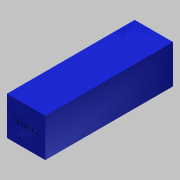
# Autodesk Inventor part: Container 2 2 5 generic
Saved by Autodesk Inventor 2015 (Build 190159000, 159)
## iProperties
Created: 2015-03-07
Part Number: Container 2 2 5 generic
Material: Generic
Document SubType Name: Modeling
Designer: Vukica
Density: 1 g/cm^3
Appearance: Blue - Wall Paint - Glossy
Author: Vukica
Autodesk Inventor part; units mm, degrees
ref_plane "YZ Plane" through (0, 0, 0) normal (1, 0, 0) x (0, 1, 0)
ref_plane "XZ Plane" through (0, 0, 0) normal (0, 1, 0) x (-1, 0, 0)
ref_plane "XY Plane" through (0, 0, 0) normal (0, 0, 1) x (1, 0, 0)
sketch "Sketch1" plane through (0, 0, 0) normal (0, 0, 1) x (1, 0, 0)
  line L0 (0, 0) -> (38.1, 0)
  line L1 (38.1, 0) -> (38.1, 38.1)
  line L2 (38.1, 38.1) -> (0, 38.1)
  line L3 (0, 38.1) -> (0, 0)
  dimension "d0" = 38.1
  dimension "d1" = 38.1
  constraints: 8 end point, 2 parallel, 1 horizontal, 1 perpendicular
  measures "d0" distance of L1.end L2.end
  measures "d1" distance of L2.end L0.start
extrude "Extrusion1" add sketch "Sketch1" along normal blind 127
sketch "Sketch2" plane through (0, 0, 127) normal (0, 0, 1) x (1, 0, 0)
  line L0 (5.3755, 22.1024) -> (51.7707, 22.1024) construction
  line L1 (51.7707, 22.1024) -> (51.7707, -10.5224) construction
  line L2 (51.7707, -10.5224) -> (5.3755, -10.5224) construction
  line L3 (5.3755, -10.5224) -> (5.3755, 22.1024) construction
  spline S0 degree 2 poles (8.0184, 16.8331) (7.4792, 16.8331) (6.5858, 17.1624) (6.2647, 17.4959) knots 0 0 0 1 2 2 2
  spline S1 degree 2 poles (6.2647, 17.4959) (5.9436, 17.8334) (5.6019, 18.8297) (5.6019, 19.476) knots 0 0 0 1 2 2 2
  spline S2 degree 2 poles (5.6019, 19.476) (5.6019, 20.0894) (5.9478, 21.0609) (6.2689, 21.4067) knots 0 0 0 1 2 2 2
  spline S3 degree 2 poles (6.2689, 21.4067) (6.5776, 21.7402) (7.4833, 22.1024) (8.0226, 22.1024) knots 0 0 0 1 2 2 2
  spline S4 degree 2 poles (8.0226, 22.1024) (8.2819, 22.1024) (8.7512, 22.0283) (8.9653, 21.9625) knots 0 0 0 1 2 2 2
  spline S5 degree 2 poles (8.9653, 21.9625) (9.1382, 21.9131) (9.5581, 21.7319) (9.6857, 21.6661) knots 0 0 0 1 2 2 2
  line L4 (9.6857, 21.6661) -> (9.6857, 20.851)
  line L5 (9.6857, 20.851) -> (9.6281, 20.851)
  spline S6 degree 2 poles (9.6281, 20.851) (9.5005, 20.9621) (9.2329, 21.1638) (8.9859, 21.2791) knots 0 0 0 1 2 2 2
  spline S7 degree 2 poles (8.9859, 21.2791) (8.78, 21.382) (8.249, 21.5179) (7.9443, 21.5179) knots 0 0 0 1 2 2 2
  spline S8 degree 2 poles (7.9443, 21.5179) (7.2116, 21.5179) (6.3059, 20.4146) (6.3059, 19.4966) knots 0 0 0 1 2 2 2
  spline S9 degree 2 poles (6.3059, 19.4966) (6.3059, 18.9861) (6.5447, 18.2204) (6.7711, 17.9569) knots 0 0 0 1 2 2 2
  spline S10 degree 2 poles (6.7711, 17.9569) (6.9893, 17.6935) (7.6068, 17.4176) (7.9937, 17.4176) knots 0 0 0 1 2 2 2
  spline S11 degree 2 poles (7.9937, 17.4176) (8.2778, 17.4176) (8.8459, 17.5) (9.0394, 17.5823) knots 0 0 0 1 2 2 2
  line L6 (9.0394, 17.5823) -> (9.0394, 18.8955)
  line L7 (9.0394, 18.8955) -> (7.862, 18.8955)
  line L8 (7.862, 18.8955) -> (7.862, 19.4883)
  line L9 (7.862, 19.4883) -> (9.7063, 19.4883)
  line L10 (9.7063, 19.4883) -> (9.7063, 17.2694)
  spline S12 degree 2 poles (9.7063, 17.2694) (9.5787, 17.2118) (9.1423, 17.0348) (8.9571, 16.9813) knots 0 0 0 1 2 2 2
  spline S13 degree 2 poles (8.9571, 16.9813) (8.7059, 16.9072) (8.3025, 16.8331) (8.0184, 16.8331) knots 0 0 0 1 2 2 2
  line L11 (10.5543, 16.9319) -> (10.5543, 22.0119)
  line L12 (10.5543, 22.0119) -> (13.7324, 22.0119)
  line L13 (13.7324, 22.0119) -> (13.7324, 21.4108)
  line L14 (13.7324, 21.4108) -> (11.2295, 21.4108)
  line L15 (11.2295, 21.4108) -> (11.2295, 20.0194)
  line L16 (11.2295, 20.0194) -> (13.5636, 20.0194)
  line L17 (13.5636, 20.0194) -> (13.5636, 19.4184)
  line L18 (13.5636, 19.4184) -> (11.2295, 19.4184)
  line L19 (11.2295, 19.4184) -> (11.2295, 17.5329)
  line L20 (11.2295, 17.5329) -> (13.7324, 17.5329)
  line L21 (13.7324, 17.5329) -> (13.7324, 16.9319)
  line L22 (13.7324, 16.9319) -> (10.5543, 16.9319)
  line L23 (18.1085, 16.9319) -> (17.351, 16.9319)
  line L24 (17.351, 16.9319) -> (15.1033, 21.312)
  line L25 (15.1033, 21.312) -> (15.1033, 16.9319)
  line L26 (15.1033, 16.9319) -> (14.4734, 16.9319)
  line L27 (14.4734, 16.9319) -> (14.4734, 22.0119)
  line L28 (14.4734, 22.0119) -> (15.4326, 22.0119)
  line L29 (15.4326, 22.0119) -> (17.4786, 17.9899)
  line L30 (17.4786, 17.9899) -> (17.4786, 22.0119)
  line L31 (17.4786, 22.0119) -> (18.1085, 22.0119)
  line L32 (18.1085, 22.0119) -> (18.1085, 16.9319)
  line L33 (19.1376, 16.9319) -> (19.1376, 22.0119)
  line L34 (19.1376, 22.0119) -> (22.3157, 22.0119)
  line L35 (22.3157, 22.0119) -> (22.3157, 21.4108)
  line L36 (22.3157, 21.4108) -> (19.8128, 21.4108)
  line L37 (19.8128, 21.4108) -> (19.8128, 20.0194)
  line L38 (19.8128, 20.0194) -> (22.1469, 20.0194)
  line L39 (22.1469, 20.0194) -> (22.1469, 19.4184)
  line L40 (22.1469, 19.4184) -> (19.8128, 19.4184)
  line L41 (19.8128, 19.4184) -> (19.8128, 17.5329)
  line L42 (19.8128, 17.5329) -> (22.3157, 17.5329)
  line L43 (22.3157, 17.5329) -> (22.3157, 16.9319)
  line L44 (22.3157, 16.9319) -> (19.1376, 16.9319)
  line L45 (26.9882, 16.9319) -> (26.1113, 16.9319)
  line L46 (26.1113, 16.9319) -> (24.5058, 18.9532)
  line L47 (24.5058, 18.9532) -> (23.7319, 18.9532)
  line L48 (23.7319, 18.9532) -> (23.7319, 16.9319)
  line L49 (23.7319, 16.9319) -> (23.0567, 16.9319)
  line L50 (23.0567, 16.9319) -> (23.0567, 22.0119)
  line L51 (23.0567, 22.0119) -> (24.3658, 22.0119)
  spline S14 degree 2 poles (24.3658, 22.0119) (24.8022, 22.0119) (25.3909, 21.9172) (25.6585, 21.7443) knots 0 0 0 1 2 2 2
  spline S15 degree 2 poles (25.6585, 21.7443) (25.9261, 21.5714) (26.2348, 21.0321) (26.2348, 20.6328) knots 0 0 0 1 2 2 2
  spline S16 degree 2 poles (26.2348, 20.6328) (26.2348, 20.077) (25.6667, 19.3237) (25.1809, 19.1425) knots 0 0 0 1 2 2 2
  line L52 (25.1809, 19.1425) -> (26.9882, 16.9319)
  spline S17 degree 2 poles (25.5309, 20.5793) (25.5309, 20.8016) (25.3744, 21.1432) (25.2098, 21.2544) knots 0 0 0 1 2 2 2
  spline S18 degree 2 poles (25.2098, 21.2544) (25.0657, 21.3491) (24.6828, 21.4273) (24.4029, 21.4273) knots 0 0 0 1 2 2 2
  line L53 (24.4029, 21.4273) -> (23.7319, 21.4273)
  line L54 (23.7319, 21.4273) -> (23.7319, 19.5172)
  line L55 (23.7319, 19.5172) -> (24.3247, 19.5172)
  spline S19 degree 2 poles (24.3247, 19.5172) (24.617, 19.5172) (25.0821, 19.6201) (25.2427, 19.7806) knots 0 0 0 1 2 2 2
  spline S20 degree 2 poles (25.2427, 19.7806) (25.3909, 19.9206) (25.5309, 20.3158) (25.5309, 20.5793) knots 0 0 0 1 2 2 2
  line L56 (29.1618, 16.9319) -> (27.194, 16.9319)
  line L57 (27.194, 16.9319) -> (27.194, 17.4506)
  line L58 (27.194, 17.4506) -> (27.8403, 17.4506)
  line L59 (27.8403, 17.4506) -> (27.8403, 21.4932)
  line L60 (27.8403, 21.4932) -> (27.194, 21.4932)
  line L61 (27.194, 21.4932) -> (27.194, 22.0119)
  line L62 (27.194, 22.0119) -> (29.1618, 22.0119)
  line L63 (29.1618, 22.0119) -> (29.1618, 21.4932)
  line L64 (29.1618, 21.4932) -> (28.5155, 21.4932)
  line L65 (28.5155, 21.4932) -> (28.5155, 17.4506)
  line L66 (28.5155, 17.4506) -> (29.1618, 17.4506)
  line L67 (29.1618, 17.4506) -> (29.1618, 16.9319)
  spline S21 degree 2 poles (31.9817, 16.8413) (31.4877, 16.8413) (30.652, 17.1748) (30.3474, 17.5082) knots 0 0 0 1 2 2 2
  spline S22 degree 2 poles (30.3474, 17.5082) (30.0428, 17.8375) (29.7093, 18.8255) (29.7093, 19.4678) knots 0 0 0 1 2 2 2
  spline S23 degree 2 poles (29.7093, 19.4678) (29.7093, 20.1058) (30.0345, 21.0527) (30.3433, 21.4026) knots 0 0 0 1 2 2 2
  spline S24 degree 2 poles (30.3433, 21.4026) (30.6479, 21.7443) (31.4795, 22.1024) (31.9941, 22.1024) knots 0 0 0 1 2 2 2
  spline S25 degree 2 poles (31.9941, 22.1024) (32.2493, 22.1024) (32.698, 22.0283) (32.8874, 21.9707) knots 0 0 0 1 2 2 2
  spline S26 degree 2 poles (32.8874, 21.9707) (33.0521, 21.9172) (33.3937, 21.7649) (33.5625, 21.6743) knots 0 0 0 1 2 2 2
  line L68 (33.5625, 21.6743) -> (33.5625, 20.8592)
  line L69 (33.5625, 20.8592) -> (33.509, 20.8592)
  spline S27 degree 2 poles (33.509, 20.8592) (33.4184, 20.9415) (33.1385, 21.1721) (32.9368, 21.2832) knots 0 0 0 1 2 2 2
  spline S28 degree 2 poles (32.9368, 21.2832) (32.7433, 21.3902) (32.2864, 21.5261) (31.99, 21.5261) knots 0 0 0 1 2 2 2
  spline S29 degree 2 poles (31.99, 21.5261) (31.6647, 21.5261) (31.0843, 21.2585) (30.8661, 21.0033) knots 0 0 0 1 2 2 2
  spline S30 degree 2 poles (30.8661, 21.0033) (30.652, 20.7439) (30.4133, 19.9576) (30.4133, 19.4678) knots 0 0 0 1 2 2 2
  spline S31 degree 2 poles (30.4133, 19.4678) (30.4133, 18.9449) (30.6644, 18.1916) (30.8826, 17.9322) knots 0 0 0 1 2 2 2
  spline S32 degree 2 poles (30.8826, 17.9322) (31.0966, 17.6811) (31.6689, 17.4259) (31.99, 17.4259) knots 0 0 0 1 2 2 2
  spline S33 degree 2 poles (31.99, 17.4259) (32.2822, 17.4259) (32.7804, 17.57) (32.9738, 17.677) knots 0 0 0 1 2 2 2
  spline S34 degree 2 poles (32.9738, 17.677) (33.1591, 17.784) (33.4349, 18.0063) (33.5131, 18.0845) knots 0 0 0 1 2 2 2
  line L70 (33.5131, 18.0845) -> (33.5625, 18.0845)
  line L71 (33.5625, 18.0845) -> (33.5625, 17.2777)
  spline S35 degree 2 poles (33.5625, 17.2777) (33.3937, 17.1995) (33.0973, 17.0554) (32.8874, 16.9895) knots 0 0 0 1 2 2 2
  spline S36 degree 2 poles (32.8874, 16.9895) (32.6651, 16.9154) (32.2864, 16.8413) (31.9817, 16.8413) knots 0 0 0 1 2 2 2
  point P0 (0, 0)
  constraints: 2 other
extrude "Extrusion3" cut sketch "Sketch2" against normal blind 0.254
equation "\"d1\" = d0"
body "Solid1"
